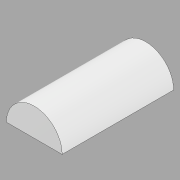
# Autodesk Inventor part: Greenhouse
Saved by Autodesk Inventor 2022 (Build 260153000, 153)
## iProperties
Created: 2021-09-02
Part Number: Greenhouse
Material: Generic
Document SubType Name: Modeling
Designer: Ben
Density: 1 g/cm^3
Appearance: Smooth - White
Author: Ben
## iProperties of the stored document Greenhouse_3DPrint.ipt
Created: 2021-09-02
Part Number: Greenhouse_3DPrint
Material: Generic
Document SubType Name: Modeling
Designer: Ben
Density: 1 g/cm^3
Appearance: Default
Author: Ben
Autodesk Inventor part; units mm, degrees
ref_plane "YZ Plane" through (0, 0, 0) normal (1, 0, 0) x (0, 1, 0)
ref_plane "XZ Plane" through (0, 0, 0) normal (0, 1, 0) x (-1, 0, 0)
ref_plane "XY Plane" through (0, 0, 0) normal (0, 0, 1) x (1, 0, 0)
sketch "Sketch1" plane through (0, 0, 0) normal (0, 0, 1) x (1, 0, 0)
  arc A0 (31.75, 0) -> (-31.75, 0) centre (0, 0) ccw
  line L0 (-31.75, 0) -> (31.75, 0)
  dimension "diameter" = 63.5
  constraints: 2 end point, 2 point on circle, 1 centre point, 1 coincident, 1 horizontal
  measures "diameter" diameter of A0
extrude "Extrusion1" add sketch "Sketch1" along normal blind 127
sketch "Sketch2" plane through (-31.75, 0, 0) normal (0, -1, 0) x (1, 0, 0)
  line L0 (31.75, 0) -> (31.75, 127) construction
  line L1 (0, 127) -> (63.5, 127) construction
  line L2 (0, 0) -> (0, 127) construction
  line L3 (0, 63.5) -> (63.5, 63.5) construction
  line L4 (63.5, 0) -> (63.5, 127) construction
  point P0 (31.75, 63.5)
  point P1 (31.75, 107.95)
  point P2 (31.75, 19.05)
  point P3 (47.625, 63.5)
  point P4 (15.875, 63.5)
  dimension "d3" = 44.45
  dimension "d4" = 44.45
  dimension "d12" = 15.875
  constraints: 4 end point, 4 midpoint, 3 point on line, 1 symmetric about line
  measures "d3" distance of point (31.75, 107.95) point (31.75, 63.5)
  measures "d4" distance of point (31.75, 19.05) point (31.75, 63.5)
  measures "d12" distance of point (47.625, 63.5) point (31.75, 63.5)
hole "Hole1" at (0, 0, 107.95) at (0, 0, 19.05) at (15.875, 0, 63.5) at (-15.875, 0, 63.5) direction (0, 1, 0) diameter 4.7625 depth 6.35
hole "Hole2" at (0, 0, 63.5) direction (0, 1, 0) diameter 7.9375 depth 12.7
equation "\"width\" = 2 * diameter"
equation "\"d4\" = d3"
body "Solid1"
